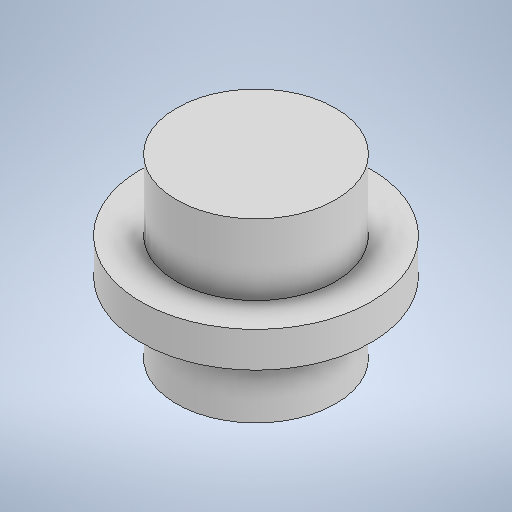
# Autodesk Inventor part: Part5
Saved by Autodesk Inventor 2025.2 (Build 292293000, 293)
## iProperties
Created: 2025-06-06
Part Number: Part5
Material: Generic
Document SubType Name: Sheet Metal
Designer: ziyuz
Density: 1 g/cm^3
Sheet Metal Rule: Default_mm
Appearance: Default
Author: ziyuz
Autodesk Inventor part; units mm, degrees
ref_plane "YZ Plane" through (0, 0, 0) normal (1, 0, 0) x (0, 1, 0)
ref_plane "XZ Plane" through (0, 0, 0) normal (0, 1, 0) x (-1, 0, 0)
ref_plane "XY Plane" through (0, 0, 0) normal (0, 0, 1) x (1, 0, 0)
sketch "Sketch1" plane through (0, 0, 0) normal (0, 1, 0) x (-1, 0, 0)
  circle A0 centre (0, 0) radius 3.25
  dimension "d0" = 6.5
  constraints: 1 centre point, 1 coincident
  measures "d0" diameter of A0
extrude "Extrusion1" add sketch "Sketch1" along normal blind 1
sketch "Sketch2" plane through (0, 1, 0) normal (0, 1, 0) x (1, 0, 0)
  circle A0 centre (0, 0) radius 2.25
  dimension "d3" = 4.5
  constraints: 1 centre point, 1 coincident
  measures "d3" diameter of A0
extrude "Extrusion2" add sketch "Sketch2" along normal blind 2
sketch "Sketch3" plane through (0, 0, 0) normal (0, -1, 0) x (1, 0, 0)
  circle A0 centre (0, 0) radius 2.25
  constraints: 1 centre point, 1 coincident
extrude "Extrusion3" add sketch "Sketch3" along normal blind 2
equation "\"BendRadius\" = Thickness"
equation "\"BendReliefWidth\" = Thickness"
equation "\"BendReliefDepth\" = 0.5 * Thickness"
equation "\"CornerReliefSize\" = 4 * Thickness"
equation "\"MinimumRemnant\" = 2 * Thickness"
equation "\"TransitionRadius\" = BendRadius"
equation "\"JacobiRadiusSize\" = BendRadius"
equation "\"GapSize\" = Thickness"
equation "\"Thickness\" = 0.5"
body "Solid1"
